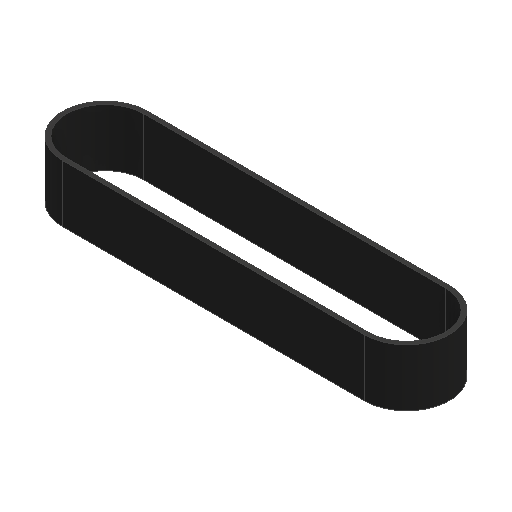
# Autodesk Inventor part: COTS_GENERIC_Y_Axis_GT2_Timing_Belt_Stepper
Saved by Autodesk Inventor 2026.1 (Build 301233000, 233)
## iProperties
Created: 2016-06-17
Part Number: COTS_GENERIC_Y_Axis_GT2_Timing_Belt_Stepper
Material: Ogólny
Document SubType Name: Modeling
Designer: Andrzej
Density: 1 g/cm^3
Appearance: Kauczuk - czarny
Mass: 0.789301 g
Surface Area: 26.0402 cm^2
Volume: 0.789301 cm^3
Author: Andrzej
Autodesk Inventor part; units mm, degrees
ref_plane "YZ Plane" through (0, 0, 0) normal (1, 0, 0) x (0, 1, 0)
ref_plane "XZ Plane" through (0, 0, 0) normal (0, 1, 0) x (-1, 0, 0)
ref_plane "XY Plane" through (0, 0, 0) normal (0, 0, 1) x (1, 0, 0)
sketch "Szkic1" plane through (0, 0, 0) normal (0, 0, 1) x (1, 0, 0)
  line L0 (-14.4483, 0) -> (32.9857, 0) construction
  line L1 (-14.4483, -6.05) -> (32.9857, -6.05)
  line L2 (32.9857, 6.05) -> (-14.4483, 6.05)
  arc A0 (-14.4483, 6.05) -> (-14.4483, -6.05) centre (-14.4483, 0) ccw
  arc A1 (32.9857, -6.05) -> (32.9857, 6.05) centre (32.9857, 0) ccw
  line L3 (-14.4483, 6.7) -> (32.9857, 6.7)
  arc A2 (32.9857, -6.7) -> (32.9857, 6.7) centre (32.9857, 0) ccw
  line L4 (32.9857, -6.7) -> (-14.4483, -6.7)
  arc A3 (-14.4483, 6.7) -> (-14.4483, -6.7) centre (-14.4483, 0) ccw
  point P0 (0, 0)
  point P1 (9.2687, 0)
  dimension "d0" = 47.434
  dimension "d1" = 12.1
  dimension "d2" = 0.65
  constraints: 12 end point, 8 point on circle, 4 centre point, 4 tangent, 2 parallel, 1 horizontal, 1 midpoint, 3 other
  measures "d0" distance of L0.start L0.end
  measures "d1" diameter of A1
  measures "d2" distance between parallel lines of L2 L3
extrude "Wyciągnięcie proste1" add sketch "Szkic1" along normal blind 9
